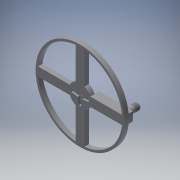
# Autodesk Inventor part: Ruedaprincipal
Saved by Autodesk Inventor 2016 (Build 200138000, 138)
## iProperties
Created: 2020-03-18
Part Number: Ruedaprincipal
Material: Genérico
Document SubType Name: Modeling
Designer: Andres Gomez
Density: 1 g/cm^3
Appearance: Valor por defecto
Author: Andres Gomez
Autodesk Inventor part; units mm, degrees
ref_plane "YZ Plane" through (0, 0, 0) normal (1, 0, 0) x (0, 1, 0)
ref_plane "XZ Plane" through (0, 0, 0) normal (0, 1, 0) x (-1, 0, 0)
ref_plane "XY Plane" through (0, 0, 0) normal (0, 0, 1) x (1, 0, 0)
sketch "Boceto1" plane through (0, 0, 0) normal (0, 1, 0) x (-1, 0, 0)
  circle A0 centre (0.4775, 1.7223) radius 65
  circle A1 centre (0.4775, 1.7223) radius 25
  circle A2 centre (0.4775, 1.7223) radius 62.5
  line L0 (0.4775, 1.7223) -> (0.4775, -20.2777)
  line L1 (0.4775, -20.2777) -> (10.4775, -20.2777)
  line L2 (10.4775, -20.2777) -> (-9.5225, -20.2777)
  line L3 (-9.5225, -20.2777) -> (-9.5225, -62.2777)
  line L4 (-9.5225, -62.2777) -> (10.4763, -62.504)
  line L5 (10.4775, -20.2777) -> (10.4775, -62.2777)
  line L6 (0.4775, 1.7223) -> (-21.5225, 1.7223)
  line L7 (-21.5225, 1.7223) -> (-21.5225, -8.2777)
  line L8 (-21.5225, 1.7223) -> (-11.5225, 1.7223) construction
  line L9 (-21.5225, -8.2777) -> (-21.5225, 11.7223)
  line L10 (-21.5225, 11.7223) -> (-63.5225, 11.7223)
  line L11 (-63.5225, 11.7223) -> (-63.5225, -8.2777)
  line L12 (-63.5225, -8.2777) -> (-21.5225, -8.2777)
  line L13 (0.4775, 1.7223) -> (0.4775, 23.7223)
  line L14 (0.4775, 1.7223) -> (22.4775, 1.7223) construction
  line L15 (0.4775, 23.7223) -> (10.4775, 23.7223)
  line L16 (10.4775, 23.7223) -> (-9.5225, 23.7223)
  line L17 (-9.5225, 23.7223) -> (-9.5225, 65.7223)
  line L18 (-9.5225, 65.7223) -> (10.4775, 65.7223)
  line L19 (10.4775, 23.7223) -> (10.4775, 65.7223)
  line L20 (10.4775, 23.7223) -> (52.4775, 23.7223) construction
  line L21 (0.4775, 1.7223) -> (22.4775, 1.7223)
  line L22 (22.4775, 1.7223) -> (22.4775, -8.2777)
  line L23 (22.4775, -8.2777) -> (22.4775, 11.7223)
  line L24 (22.4775, 11.7223) -> (64.4775, 11.7223)
  line L25 (64.4775, 11.7223) -> (64.4775, -8.2777)
  line L26 (64.4775, -8.2777) -> (22.4775, -8.2777)
  line L27 (10.4775, -62.2777) -> (-9.5225, -62.2777)
  line L28 (-9.5225, -62.2777) -> (-9.5225, -20.2777)
  line L29 (-9.5225, -20.2777) -> (10.4775, -20.2777)
  line L30 (10.4775, -20.2777) -> (10.4775, -62.2777)
  dimension "d57" = 130
  dimension "d58" = 50
  dimension "d59" = 125
  dimension "d60" = 22
  dimension "d61" = 10
  dimension "d62" = 20
  dimension "d63" = 42
  dimension "d64" = 20
  dimension "d65" = 42
  dimension "d66" = 22
  dimension "d67" = 10
  dimension "d68" = 90
  dimension "d69" = 20
  dimension "d70" = 0
  dimension "d71" = 42
  dimension "d72" = 20
  dimension "d73" = 90
  dimension "d74" = 22
  dimension "d75" = 90
  dimension "d76" = 10
  dimension "d77" = 90
  dimension "d78" = 20
  dimension "d79" = 42
  dimension "d80" = 90
  dimension "d81" = 20
  dimension "d82" = 90
  dimension "d83" = 42
  dimension "d84" = 90
  dimension "d85" = 22
  dimension "d86" = 10
  dimension "d87" = 90
  dimension "d88" = 20
  dimension "d89" = 42
  dimension "d90" = 90
  dimension "d91" = 20
  dimension "d92" = 90
  constraints: 62 end point, 14 perpendicular, 6 horizontal, 3 point on line, 3 vertical, 2 centre point, 2 coincident, 2 collinear, 2 parallel, 3 other
  measures "d58" diameter of A1
  measures "d59" diameter of A2
  measures "d60" distance of L0.start L0.end
  measures "d61" distance of L0.end L1.end
  measures "d62" distance of L1.end L2.end
  measures "d63" distance of L2.end L3.end
  measures "d64" distance of L3.end L4.end
  measures "d65" distance of L1.end L5.end
  measures "d66" distance of L0.start L6.end
  measures "d67" distance of L6.end L7.end
  measures "d68" angle of L7 L8
  measures "d69" distance of L7.end L9.end
  measures "d70" distance between parallel lines of L9 L7
  measures "d71" distance of L9.end L10.end
  measures "d72" distance of L10.end L11.end
  measures "d73" angle of L11 L10
  measures "d74" distance of L0.start L13.end
  measures "d75" angle of L14 L13
  measures "d76" distance of L13.end L15.end
  measures "d77" angle of L13 L15
  measures "d78" distance of L15.end L16.end
  measures "d79" distance of L16.end L17.end
  measures "d80" angle of L16 L17
  measures "d81" distance of L17.end L18.end
  measures "d82" angle of L17 L18
  measures "d83" distance of L15.end L18.end
  measures "d84" angle of L20 L19
  measures "d85" distance of L0.start L14.end
  measures "d86" distance of L14.end L22.end
  measures "d87" angle of L21 L22
  measures "d88" distance of L22.end L23.end
  measures "d89" distance of L23.end L24.end
  measures "d90" angle of L23 L24
  measures "d91" distance of L24.end L25.end
  measures "d92" angle of L24 L25
ref_plane "Plano de trabajo1" through (0, 10, 0) normal (0, 1, 0) x (1, 0, 0)
extrude "Extrusión10" add sketch "Boceto1" along normal blind 7 contours A0 | A1 L26 L22 L23 L24 | A1 L24 A2 L26 | L24 L23 L21 L13 L15 L19 A1 | A1 L5 L1 L0 L21 L22 L26 | L19 L15 L16 L17 A1 | A1 L17 A2 L19 | L24 L25 L26 A2 | L5 A2 L3 A1 | A1 L3 L2 L1 L5 | L17 L16 L13 L6 L9 L10 A1 | A2 L17 L18 L19 | A1 L12 L7 L6 L0 L2 L3 | L5 L27 L3 A2 | L10 L9 L7 L12 A1 | A1 L12 A2 L10 | A2 L12 L11 L10
sketch "Boceto13" plane through (-0.4775, 7, 1.7223) normal (0, 1, 0) x (1, 0, 0)
  circle A0 centre (0, 0) radius 65 projected
  line L0 (36.201, 9.9521) -> (64.2042, 9.9521)
  line L1 (64.2042, 9.9521) -> (64.2042, -10.1398)
  line L2 (64.2042, -10.1398) -> (36.201, -10.1398)
  line L3 (36.201, -10.1398) -> (36.201, 9.9521)
  point P0 (0.4775, 1.7223)
  constraints: 8 end point, 2 parallel, 1 horizontal, 1 perpendicular, 2 other
extrude "Extrusión13" add sketch "Boceto13" along normal blind 10 contours L2 L3 L0 L1
sketch "Boceto14" plane through (0, 7, 0) normal (0, 1, 0) x (1, 0, 0)
  circle A0 centre (-0.4775, -1.7223) radius 65 projected
  arc A1 (63.7267, -11.8621) -> (63.7267, 8.4174) centre (-0.4775, -1.7223) ccw
  line L0 (63.7267, 8.4174) -> (63.7267, -11.8621)
  point P0 (0, 0)
  constraints: 3 point on circle, 2 end point, 1 centre point, 1 vertical
extrude "Extrusión14" add sketch "Boceto14" along normal blind 10 contours A0 L0 picked at (63.874, 0.5361)
sketch "Boceto16" plane through (-0.4775, 17, 1.7223) normal (0, 1, 0) x (1, 0, 0)
  line L0 (62.5013, -7.7985) -> (47.0013, -7.7985)
  line L1 (47.0013, -7.7985) -> (47.0013, 7.7015)
  line L2 (47.0013, 7.7015) -> (62.5013, 7.7015)
  line L3 (62.5013, 7.7015) -> (62.5013, -7.7985)
  line L4 (62.5013, -7.7985) -> (47.0013, 7.7015) construction
  line L5 (47.0013, -7.7985) -> (62.5013, 7.7015) construction
  point P0 (0.4775, 1.7223)
  dimension "d106" = 15.5
  dimension "d107" = 15.5
  constraints: 12 end point, 2 parallel, 1 horizontal, 1 perpendicular
  measures "d106" distance of L1.end L2.end
  measures "d107" distance of L0.end L1.end
extrude "Extrusión15" add sketch "Boceto16" along normal blind 2
sketch "Boceto17" plane through (-0.4775, 19, 1.7223) normal (0, 1, 0) x (1, 0, 0)
  circle A0 centre (54.8827, -0.0485) radius 7.4
  point P0 (0.4775, 1.7223)
  dimension "d110" = 14.8
  constraints: 1 centre point
  measures "d110" diameter of A0
extrude "Extrusión16" add sketch "Boceto17" along normal blind 30
sketch "Boceto18" plane through (-0.4775, 0, 1.7223) normal (0, -1, 0) x (1, 0, 0)
  circle A0 centre (0, 0) radius 3
  point P0 (0.4775, -1.7223)
  dimension "d114" = 6
  constraints: 1 centre point
  measures "d114" diameter of A0
extrude "Extrusión17" cut sketch "Boceto18" against normal blind 30
sketch "Boceto19" plane through (-0.4775, 0, 1.7223) normal (0, -1, 0) x (1, 0, 0)
  circle A0 centre (0, 0) radius 1.5
  line L0 (4.8775, -4.6661) -> (-4.8775, 4.6661) construction
  line L1 (-4.8775, -4.6661) -> (4.8775, 4.6661) construction
  line L2 (-4.8775, 4.6661) -> (-2.7009, 19.5073)
  line L3 (4.8775, 4.6661) -> (2.7009, 19.5073)
  line L4 (2.7009, 19.5073) -> (-2.7009, 19.5073)
  line L5 (-19.7188, -2.4895) -> (-19.7188, 2.4895)
  line L6 (4.8775, -4.6661) -> (19.7188, -2.4895)
  line L7 (4.8775, 4.6661) -> (19.7188, 2.4895)
  line L8 (19.7188, 2.4895) -> (19.7188, -2.4895)
  line L9 (-2.7009, -19.5073) -> (2.7009, -19.5073)
  line L10 (-4.8775, -4.6661) -> (-2.7009, -19.5073)
  line L11 (2.7009, -19.5073) -> (4.8775, -4.6661)
  line L12 (-4.8775, -4.6661) -> (4.8775, -4.6661)
  line L13 (4.8775, -4.6661) -> (4.8775, 4.6661)
  line L14 (4.8775, 4.6661) -> (-4.8775, 4.6661)
  line L15 (-4.8775, 4.6661) -> (-4.8775, -4.6661)
  line L16 (-4.8775, 4.6661) -> (-19.7188, 2.4895)
  line L17 (-4.8775, -4.6661) -> (-19.7188, -2.4895)
  dimension "d118" = 15
  dimension "d119" = 15
  dimension "d120" = 15
  dimension "d121" = 15
  dimension "d122" = 15
  constraints: 36 end point, 3 perpendicular, 2 horizontal, 2 midpoint, 2 vertical, 1 centre point
  measures "d118" distance of L0.end L2.end
  measures "d119" distance of L1.end L3.end
  measures "d120" distance of L0.end L5.end
  measures "d121" distance of L1.start L5.start
  measures "d122" distance of L0.start L6.end
extrude "Extrusión18" cut sketch "Boceto19" against normal blind 3
sketch "Boceto20" plane through (-0.4775, 3, 1.7223) normal (0, -1, 0) x (1, 0, 0)
  circle A0 centre (-9.5726, 0) radius 1
  circle A1 centre (0, 0) radius 3 projected
  circle A2 centre (9.3899, 0) radius 1
  circle A3 centre (0, -8.454) radius 1
  circle A4 centre (0, 8.4227) radius 1
  circle A5 centre (-13.7812, 0) radius 1
  circle A6 centre (14.3966, 0) radius 1
  circle A7 centre (0, -12.6971) radius 1
  circle A8 centre (0, 13.551) radius 1
  point P0 (0.4775, -1.7223)
  dimension "d125" = 2
  dimension "d127" = 2
  dimension "d128" = 2
  dimension "d129" = 2
  dimension "d130" = 2
  dimension "d131" = 2
  dimension "d132" = 2
  dimension "d133" = 2
  constraints: 8 centre point
  measures "d125" diameter of A0
  measures "d127" diameter of A2
  measures "d128" diameter of A3
  measures "d129" diameter of A4
  measures "d130" diameter of A5
  measures "d131" diameter of A6
  measures "d132" diameter of A7
  measures "d133" diameter of A8
extrude "Extrusión19" cut sketch "Boceto20" against normal blind 7 contours A0 | A2 | A3 | A4 | A5 | A6 | A7 | A8
sketch "Boceto21" plane through (-0.4775, 3, 1.7223) normal (0, -1, 0) x (1, 0, 0)
  circle A0 centre (0, 0) radius 3.5
  point P0 (0.4775, -1.7223)
  dimension "d136" = 7
  constraints: 1 centre point
  measures "d136" diameter of A0
extrude "Extrusión20" add sketch "Boceto21" against normal blind 3
sketch "Boceto22" plane through (-0.4775, 3, 1.7223) normal (0, -1, 0) x (1, 0, 0)
  circle A0 centre (0, 0) radius 1.5
  point P0 (0.4775, -1.7223)
  dimension "d139" = 3
  constraints: 1 centre point
  measures "d139" diameter of A0
extrude "Extrusión21" cut sketch "Boceto22" against normal blind 7
fillet "Empalme5" radius 0.5 4 edges at (46.5238, 19, 1.7709) (54.2738, 19, 9.5209) (54.2738, 19, -5.9791) (62.0238, 19, 1.7709)
fillet "Empalme6" radius 1 8 edges at (62.0238, 17.75, -5.9791) (61.8773, 18.8536, -5.8327) (46.5238, 17.75, -5.9791) (46.6702, 18.8536, -5.8327) (61.8773, 18.8536, 9.3744) (62.0238, 17.75, 9.5209) (46.6702, 18.8536, 9.3744) (46.5238, 17.75, 9.5209)
fillet "Empalme7" radius 1 4 edges at (63.7267, 12, -8.2298) (35.7235, 12, -8.2298) (35.7235, 12, 11.8621) (63.7267, 12, 11.8621)
thread "Rosca2" size "M15x1.5" class "6g" standard "ANSI Metric M Profile" length 13
